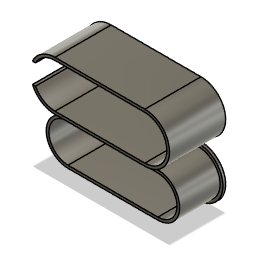
Zahnb_case (Autodesk Fusion 360 design; units mm, degrees)
Autodesk Fusion 360 part; units mm, degrees
sketch "Skizze1" plane through (0, 0, 0) normal (0, 0, 1) x (1, 0, 0)
  line L0 (20, 11) -> (-20, 11)
  arc A0 (-20, 11) -> (-20, -11) centre (-20, 0) ccw
  line L1 (-20, -11) -> (20, -11)
  arc A1 (20, -11) -> (20, 11) centre (20, 0) ccw
  line L2 (20, 0) -> (-20, 0) construction
  dimension "d1" = 40
  dimension "d2" = 11
  constraint tangent L0 A0
  constraint tangent A0 L1
  constraint parallel L0 L1
  constraint tangent L1 A1
  constraint tangent L0 A1
  constraint horizontal L2
  constraint midpoint L2 origin
  measures "d1" distance of A1.centre A0.centre
  measures "d2" radius of A1
extrude "Extrusion1" add sketch "Skizze1" along normal blind 25 makes body 1
shell "Schale1" thickness 1.2 removed faces 1 at (-6.6667, -3.6667, 25) on bodies 1
sketch "Skizze2" plane through (0, 0, 1.2) normal (0, 0, 1) x (1, 0, 0)
  arc A0 (20, -9.8) -> (20, 9.8) centre (20, 0) ccw
  line L0 (20, 9.8) -> (-20, 9.8)
  arc A1 (-20, 9.8) -> (-20, -9.8) centre (-20, 0) ccw
  line L1 (-20, -9.8) -> (20, -9.8)
  line L2 (-33, 4.5) -> (-25, 4.5)
  line L3 (-25, 4.5) -> (-25, -4.5)
  line L4 (-25, -4.5) -> (-33, -4.5)
  line L5 (-33, -4.5) -> (-33, 4.5)
  line L6 (-33, 4.5) -> (-25, -4.5) construction
  line L7 (-25, 4.5) -> (-33, -4.5) construction
  point P0 (-29, 0)
  dimension "d6" = 9
  dimension "d7" = 25
  dimension "d8" = 8
  constraint horizontal L2
  constraint perpendicular L2 L3
  constraint parallel L2 L4
  constraint parallel L3 L5
  constraint coincident L6 P0
  constraint coincident L7 P0
  constraint horizontal origin P0
  measures "d6" distance of L2.end L3.end
  measures "d7" distance of origin L3
  measures "d8" distance of L2.start L2.end
extrude "Extrusion2" cut sketch "Skizze2" along normal blind 27 contours A1 L2 L4 L5 | A1 L2 L3 L4 bodies 1
sketch "Skizze3" plane through (0, 0, 0) normal (0, 0, -1) x (-1, 0, 0)
  arc A0 (-20, 11) -> (-20, -11) centre (-20, 0) ccw
  line L0 (-20, -11) -> (20, -11)
  arc A1 (20, -11) -> (20, 11) centre (20, 0) ccw
  line L1 (20, 11) -> (-20, 11)
  line L2 (20, -14) -> (-20, -14)
  arc A2 (-20, -14) -> (-20, -36) centre (-20, -25) ccw
  line L3 (-20, -36) -> (20, -36)
  arc A3 (20, -36) -> (20, -14) centre (20, -25) ccw
  line L4 (20, -25) -> (-20, -25) construction
  point P0 (0, -25)
  dimension "d11" = 25
  constraint tangent L2 A2
  constraint tangent A2 L3
  constraint parallel L2 L3
  constraint tangent L3 A3
  constraint tangent L2 A3
  constraint horizontal L4
  constraint midpoint L4 P0
  constraint equal L0 L2
  constraint equal A1 A3
  constraint vertical origin P0
  measures "d11" distance of origin L4
extrude "Extrusion3" add sketch "Skizze3" against normal blind 1.2 separate body contours L2 A2 L3 A3 makes body 2
sketch "Skizze4" plane through (0, 0, 1.2) normal (0, 0, 1) x (1, 0, 0)
  arc A0 (-20, -14) -> (-20, -36) centre (-20, -25) ccw
  line L0 (-20, -36) -> (20, -36)
  arc A1 (20, -36) -> (20, -14) centre (20, -25) ccw
  line L1 (20, -14) -> (-20, -14)
  line L2 (-20, -25) -> (20, -25)
  line L3 (-20, -34.725) -> (20, -34.725)
  arc A2 (20, -34.725) -> (20, -15.275) centre (20, -25) ccw
  line L4 (20, -15.275) -> (-20, -15.275)
  arc A3 (-20, -15.275) -> (-20, -34.725) centre (-20, -25) ccw
  line L5 (-20, -25) -> (20, -25) construction
  line L6 (-20, -33.525) -> (20, -33.525)
  arc A4 (20, -33.525) -> (20, -16.475) centre (20, -25) ccw
  line L7 (20, -16.475) -> (-20, -16.475)
  arc A5 (-20, -16.475) -> (-20, -33.525) centre (-20, -25) ccw
  line L8 (-20, -25) -> (20, -25) construction
  dimension "d14" = 19.45
  dimension "d15" = 1.2
  constraint coincident A0.centre L2.start
  constraint coincident A1.centre L2.end
  constraint tangent L3 A2
  constraint tangent A2 L4
  constraint parallel L3 L4
  constraint tangent L4 A3
  constraint tangent L3 A3
  constraint parallel L2 L5
  constraint tangent L6 A4
  constraint tangent A4 L7
  constraint parallel L6 L7
  constraint tangent L7 A5
  constraint tangent L6 A5
  constraint parallel L5 L8
  measures "d14" distance of L3 L4
  measures "d15" distance of L4 L7
extrude "Extrusion4" add sketch "Skizze4" along normal blind 18 contours L3 A2 L4 A3 bodies 2
